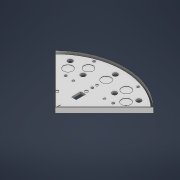
# Autodesk Inventor part: 球場2
Saved by Autodesk Inventor 2021 (Build 250183000, 183)
## iProperties
Created: 2020-12-24
Part Number: 球場2
Material: 一般
Document SubType Name: Modeling
Designer: zihon
Density: 1 g/cm^3
Appearance: 預設
Author: zihon
Autodesk Inventor part; units mm, degrees
ref_plane "YZ Plane" through (0, 0, 0) normal (1, 0, 0) x (0, 1, 0)
ref_plane "XZ Plane" through (0, 0, 0) normal (0, 1, 0) x (-1, 0, 0)
ref_plane "XY Plane" through (0, 0, 0) normal (0, 0, 1) x (1, 0, 0)
sketch "草圖1" plane through (0, 0, 0) normal (0, 1, 0) x (-1, 0, 0)
  line L0 (0, 0) -> (-1060.6602, -1060.6602)
  arc A0 (-1060.6602, -1060.6602) -> (0, -1500) centre (0, 0) ccw
  line L1 (0, -1500) -> (0, 0)
  line L2 (0, 0) -> (1060.6602, -1060.6602)
  arc A1 (0, -1500) -> (1060.6602, -1060.6602) centre (0, 0) ccw
  line L3 (1067.7254, -1060.6543) -> (0, 7.0711)
  line L4 (0, 7.0711) -> (-1067.7254, -1060.6543)
  arc A2 (-1067.7254, -1060.6543) -> (333.9619, -1467.4789) centre (0, 0) ccw
  arc A3 (333.9619, -1467.4789) -> (1067.7254, -1060.6543) centre (0, 0) ccw
  arc A4 (-1035.9114, -1035.9114) -> (332.6512, -1426.7334) centre (0, 0) ccw
  arc A5 (332.6512, -1426.7334) -> (1035.9114, -1035.9114) centre (0, 0) ccw
  line L5 (1549.2947, 0) -> (-1565.2813, 0) projected
  arc A6 (-24.7487, -24.7487) -> (24.7487, -24.7487) centre (0, 0) ccw
  line L6 (25, -130) -> (25, -70) construction
  line L7 (30, -125) -> (30, -75)
  line L8 (20, -75) -> (20, -125)
  arc A7 (20, -125) -> (30, -125) centre (25, -125) ccw
  arc A8 (30, -75) -> (20, -75) centre (25, -75) ccw
  line L9 (50, -400) -> (-50, -400)
  line L10 (-50, -400) -> (-50, -600)
  line L11 (-50, -600) -> (50, -600)
  line L12 (50, -600) -> (50, -400)
  line L13 (50, -400) -> (-50, -600) construction
  line L14 (-50, -400) -> (50, -600) construction
  point P0 (-7.0711, 0)
  point P1 (7.0711, 0)
  point P2 (24.7487, -682.358)
  point P3 (-24.7487, -682.358)
  point P4 (353.5534, -353.5534)
  point P5 (353.5534, -353.5534)
  point P6 (-353.5534, -353.5534)
  point P7 (-353.5534, -353.5534)
  point P8 (-7.0711, 0)
  point P9 (7.0711, 0)
  point P10 (25, -100)
  point P11 (0, -500)
  dimension "d0" = 1500
  dimension "d2" = 5
  dimension "d3" = 35
  dimension "d7" = 45
  dimension "d8" = 35
  dimension "d26" = 5
  dimension "d27" = 50
  dimension "d28" = 100
  dimension "d29" = 50
  dimension "d32" = 100
  dimension "d33" = 200
  dimension "d39" = 300
  constraints: 30 end point, 20 point on circle, 9 centre point, 7 point on line, 4 coincident, 4 tangent, 3 midpoint, 3 parallel, 2 vertical, 1 horizontal, 1 perpendicular, 1 symmetric about line, 4 other
  measures "d0" distance of L0.start L0.end
  measures "d2" radial gap between concentric circles of A1 A3
  measures "d3" radial gap between concentric circles of A1 A5
  measures "d7" angle of L5 L0
  measures "d8" radius of A6
  measures "d26" radius of A7
  measures "d27" distance of A8.centre A7.centre
  measures "d28" vertical distance of point (0, 0) point (25, -100)
  measures "d29" diameter of point (25, -100) L1
  measures "d32" distance of L9.start L9.end
  measures "d33" distance of L9.end L10.end
  measures "d39" distance from line of L9 point (25, -100)
extrude "擠出1" add sketch "草圖1" along normal blind 40 and the other way blind 70 contours L5 L4 L3 | L5 L3 A3 A2 L4
extrude "擠出2" add sketch "草圖1" against normal blind 40 contours A6 L1 L9 L10 L11 A4 L0 | A6 L2 A5 A4 L1 L11 L12 L9
sketch "草圖2" plane through (0, 0, 0) normal (0, 1, 0) x (-1, 0, 0)
  line L0 (353.5534, -353.5534) -> (0, -707.1068) construction
  line L1 (0, -707.1068) -> (-353.5534, -353.5534) construction
  line L2 (-353.5534, -353.5534) -> (0, 0) construction
  line L3 (0, 0) -> (353.5534, -353.5534) construction
  line L4 (0, -707.1068) -> (35.3553, -671.7514)
  line L5 (35.3553, -671.7514) -> (0, -636.3961)
  line L6 (0, -636.3961) -> (-35.3553, -671.7514)
  line L7 (-35.3553, -671.7514) -> (0, -707.1068)
  line L8 (318.1981, -388.9087) -> (353.5534, -353.5534)
  line L9 (353.5534, -353.5534) -> (318.1981, -318.1981)
  line L10 (318.1981, -318.1981) -> (282.8427, -353.5534)
  line L11 (282.8427, -353.5534) -> (318.1981, -388.9087)
  line L12 (-318.1981, -388.9087) -> (-282.8427, -353.5534)
  line L13 (-282.8427, -353.5534) -> (-318.1981, -318.1981)
  line L14 (-318.1981, -318.1981) -> (-353.5534, -353.5534)
  line L15 (-353.5534, -353.5534) -> (-318.1981, -388.9087)
  line L16 (-1060.6602, -1060.6602) -> (0, 0) projected
  line L17 (0, 0) -> (1060.6602, -1060.6602) projected
  arc A0 (-24.7487, -24.7487) -> (24.7487, -24.7487) centre (0, 0) ccw projected
  dimension "d15" = 500
  dimension "d19" = 50
  dimension "d20" = 50
  dimension "d21" = 50
  constraints: 32 end point, 8 collinear, 8 parallel, 8 perpendicular
  measures "d15" distance of L1.end L2.end
  measures "d19" distance of L6.end L5.end
  measures "d20" distance of L10.end L9.end
  measures "d21" distance of L14.end L13.end
extrude "擠出3" cut sketch "草圖2" against normal blind 5 contours L7 L6 L5 L4 | L11 L10 L9 L8 | L13 L12 L15 L14
sketch "草圖6" plane through (0, 0, 0) normal (0, 1, 0) x (1, 0, 0)
  line L0 (0, 0) -> (1060.6602, 1060.6602) projected
  line L1 (-1067.7254, 1060.6543) -> (0, -7.0711) projected
  arc A0 (919.2388, 919.2388) -> (-922.7676, 915.6965) centre (0, 0) ccw construction
  line L2 (0, 0) -> (-1060.6602, 1060.6602) projected
  arc A1 (777.8175, 777.8175) -> (-777.8175, 777.8175) centre (0, 0) ccw construction
  arc A2 (636.3961, 636.3961) -> (-634.8813, 637.9073) centre (0, 0) ccw construction
  circle A3 centre (0, 1300) radius 50
  arc A4 (1035.9114, 1035.9114) -> (-1035.9114, 1035.9114) centre (0, 0) ccw projected
  line L3 (0, 1465) -> (0, 0) construction
  circle A5 centre (0, 1100) radius 100
  circle A6 centre (0, 900) radius 25
  circle A7 centre (-745.6494, 1064.8977) radius 50
  circle A8 centre (-630.9341, 901.0672) radius 100
  circle A9 centre (-516.2188, 737.2368) radius 25
  circle A10 centre (745.6494, 1064.8977) radius 50
  circle A11 centre (630.9341, 901.0672) radius 100
  circle A12 centre (516.2188, 737.2368) radius 25
  arc A13 (989.9495, 989.9495) -> (-993.7497, 986.1347) centre (0, 0) ccw construction
  arc A14 (848.5281, 848.5281) -> (-848.5281, 848.5281) centre (0, 0) ccw construction
  arc A15 (707.1068, 707.1068) -> (-705.4236, 708.7859) centre (0, 0) ccw construction
  line L4 (0, 0) -> (501.0595, 1376.6497) construction
  circle A16 centre (342.0201, 939.6926) radius 50
  circle A17 centre (478.8282, 1315.5697) radius 25
  circle A18 centre (410.4242, 1127.6311) radius 100
  circle A19 centre (-342.0201, 939.6926) radius 50
  circle A20 centre (-478.8282, 1315.5697) radius 25
  circle A21 centre (-410.4242, 1127.6311) radius 100
  arc A22 (565.6854, 565.6854) -> (-565.6854, 565.6854) centre (0, 0) ccw construction
  circle A23 centre (0, 800) radius 25
  circle A24 centre (-338.0946, 725.0462) radius 25
  circle A25 centre (338.0946, 725.0462) radius 25
  point P0 (0, 1100)
  dimension "d44" = 1300
  dimension "d45" = 1100
  dimension "d46" = 900
  dimension "d47" = 100
  dimension "d48" = 200
  dimension "d49" = 50
  dimension "d52" = 35
  dimension "d54" = 100
  dimension "d55" = 100
  dimension "d56" = 100
  dimension "d57" = 25
  dimension "d58" = 100
  dimension "d59" = 50
  dimension "d60" = 200
  dimension "d63" = 100
  dimension "d66" = 50
  dimension "d69" = 25
  constraints: 25 centre point, 23 point on circle, 9 point on line, 7 symmetric about line, 5 coincident, 4 end point, 1 vertical, 17 other
  measures "d44" radius of A0
  measures "d45" radius of A1
  measures "d46" radius of A2
  measures "d47" diameter of A3
  measures "d48" diameter of A5
  measures "d49" diameter of A6
  measures "d54" radial gap between concentric circles of A0 A13
  measures "d55" radial gap between concentric circles of A1 A14
  measures "d56" radial gap between concentric circles of A2 A15
  measures "d57" angle of L0 L4
  measures "d58" diameter of A16
  measures "d59" diameter of A17
  measures "d60" diameter of A18
  measures "d63" radial gap between concentric circles of A2 A22
  measures "d66" diameter of A23
extrude "擠出6" cut sketch "草圖6" against normal blind 5 contours A5 | A6 | A8 | A11 | A18 | A21 | A24 | A25
extrude "擠出7" cut sketch "草圖6" against normal through all contours A3 | A7 | A9 | A10 | A12 | A16 | A17 | A19 | A20 | A23
